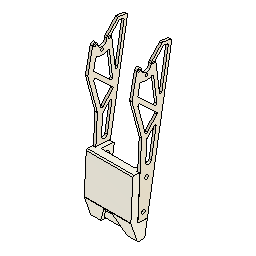
RightArm_7 (Autodesk Fusion 360 archive; units mm, degrees)
design "前腕_16"
Autodesk Fusion 360 part; units mm, degrees
sketch "スケッチ1" plane through (0, 0, 0) normal (1, 0, 0) x (0, 1, 0)
  circle A0 centre (0, 0) radius 4.025
  circle A1 centre (0, 0) radius 6 construction
  circle A2 centre (-6, 0) radius 1.025
  circle A3 centre (0, -6) radius 1.025
  circle A4 centre (6, 0) radius 1.025
  circle A5 centre (-6, 0) radius 1.975
  circle A6 centre (6, 0) radius 1.975
  arc A7 (-7.975, 0) -> (7.975, 0.000024) centre (0, 0) ccw
  line L0 (-7.040069, -110) -> (0.959931, -110)
  line L1 (0.959931, -110) -> (12.959931, -40)
  line L2 (12.959931, -40) -> (7.959931, 0.243509) construction
  circle A8 centre (0, 0) radius 10 construction
  line L3 (-7.936647, 0.387329) -> (-11.936647, -19.612671)
  line L4 (-11.936647, -19.612671) -> (-3.936647, -49.612671)
  line L5 (-3.936647, -49.612671) -> (-7.040069, -110)
  line L6 (9.714999, -38.214272) -> (4.330327, -69.624859)
  line L7 (0.409792, -52.716267) -> (-7.806231, -21.906181)
  line L8 (-7.806231, -21.906181) -> (-5.140514, -8.577594)
  line L9 (9.714999, -38.214272) -> (5.964373, -8.026597)
  arc A9 (-5.140514, -8.577594) -> (5.964373, -8.026597) centre (0, 0) ccw
  line L10 (-0.432003, -69.096168) -> (0.409792, -52.716267)
  arc A10 (-0.432003, -69.096168) -> (4.330327, -69.624859) centre (1.964834, -69.219346) ccw
  circle A11 centre (0.264062, -80) radius 5.754778 construction
  circle A12 centre (-2.400304, -104) radius 4.325705 construction
  circle A13 centre (0.264062, -80) radius 1.55
  circle A14 centre (-2.400304, -104) radius 1.55
  line L11 (12.959931, -40) -> (21.471066, 9.648289)
  line L12 (21.471066, 9.648289) -> (13.586088, 11)
  line L13 (13.586088, 11) -> (4.557732, 1.349254)
  line L14 (18.584601, 7.606643) -> (11.894088, -31.421349)
  line L15 (7.841144, 1.199587) -> (11.894088, -31.421349)
  line L16 (14.491434, 8.308329) -> (7.841144, 1.199587)
  line L17 (9.714999, -38.214272) -> (-0.505264, -49.284806)
  line L18 (8.783943, -43.645432) -> (0.409792, -52.716267)
  line L19 (9.714999, -38.214272) -> (-7.806231, -21.906181)
  line L20 (-7.115191, -18.450978) -> (9.139215, -33.579957)
  line L21 (18.584601, 7.606643) -> (14.491434, 8.308329)
  dimension "d1" = 8.05
  dimension "d2" = 12
  dimension "d3" = 2.05
  dimension "d5" = 110
  dimension "d14" = 20
  dimension "d15" = 4
  dimension "d16" = 20
  dimension "d17" = 5
  dimension "d18" = 70
  dimension "d19" = 30
  dimension "d20" = 8
  dimension "d21" = 8
  dimension "d22" = 12
  dimension "d26" = 3
  dimension "d27" = 4.5
  dimension "d28" = 3.4
  dimension "d29" = 3.5
  dimension "d30" = 4.5
  dimension "d32" = 6
  dimension "d33" = 24
  dimension "d34" = 3.1
  dimension "d35" = 8
  dimension "d36" = 11
  dimension "d38" = 2.5
  dimension "d46" = 3
  dimension "d47" = 3
  dimension "d70" = 2.5
  dimension "d72" = 2.5
  dimension "d73" = 2.4
  constraint coincident A0.centre A1.centre
  constraint concentric A0 A1
  constraint coincident A1 A2.centre
  constraint coincident A1 A3.centre
  constraint coincident A1 A4.centre
  constraint equal A3 A4
  constraint equal A2 A3
  constraint horizontal A0.centre A4.centre
  constraint horizontal A0.centre A2.centre
  constraint vertical A0.centre A3.centre
  constraint concentric A2 A5
  constraint tangent A0 A5
  constraint concentric A4 A6
  constraint tangent A0 A6
  constraint concentric A0 A7
  constraint tangent A5 A7
  constraint tangent A6 L2
  constraint coincident A5 A7.start
  constraint horizontal L0
  constraint concentric A0 A8
  constraint tangent A5 L3
  constraint parallel L2 L9
  constraint parallel L4 L7
  constraint parallel L3 L8
  constraint parallel L1 L6
  constraint parallel L5 L10
  constraint tangent L6 A10
  constraint tangent L10 A10
  constraint tangent L5 A11
  constraint tangent L1 A11
  constraint tangent L5 A12
  constraint tangent L1 A12
  constraint concentric A11 A13
  constraint concentric A12 A14
  constraint equal A13 A14
  constraint collinear L1 L11
  constraint perpendicular L11 L12
  constraint tangent A6 L13
  constraint parallel L11 L14
  constraint parallel L13 L16
  constraint parallel L17 L18
  constraint parallel L19 L20
  constraint parallel L12 L21
  measures "d1" diameter of A0
  measures "d2" diameter of A1
  measures "d3" diameter of A2
  measures "d5" distance of A0.centre L0
  measures "d14" diameter of A8
  measures "d26" distance of L2 L9
  measures "d27" distance of L3 L8
  measures "d28" distance of L4 L7
  measures "d29" distance of L1 L6
  measures "d30" distance of L5 L10
  measures "d34" diameter of A13
  measures "d38" distance of L11 L14
  measures "d46" distance of L17 L18
  measures "d47" distance of L19 L20
  measures "d70" distance of L13 L16
  measures "d72" distance of L12 L21
  measures "d73" radius of A10
extrude "押し出し1" add sketch "スケッチ1" along normal blind 2 contours A0 A5 A6 A7 | A6 | A5 | A5 A6 A7 L0 L1 L3 L4 L5 L11 L12 L13 | L8 L9 L19 L20 | L6 L7 L17 L18 picked at (-4.805093, -3.203034) picked at (7.647164, -0.149042) picked at (-7.65098, -0.098119) picked at (-4.085876, -79.829316) picked at (3.682661, -31.23347) picked at (5.997893, -43.714837) makes body 1
fillet "フィレット1" radius 1 19 edges at (1, 7.841144, 1.199587) (1, 11.894088, -31.421349) (1, 5.964373, -8.026597) (1, -5.140514, -8.577594) (1, -0.505264, -49.284806) (1, 0.409792, -52.716267) (1, 8.783943, -43.645432) (1, -11.936647, -19.612671) (1, -3.936647, -49.612671) (1, 13.586088, 11) (1, 21.471066, 9.648289) (1, 0.959931, -110) (1, -7.040069, -110) (1, 9.139215, -33.579957) (1, -7.115191, -18.450978) (1, -7.806231, -21.906181) (1, 9.714999, -38.214272) (1, 14.491434, 8.308329) (1, 18.584601, 7.606643) on bodies 1
extrude "押し出し2" add 1 faces at (2, -8.409318, -9.624556) along direction (1, 0, 0) blind 2 from surface at 35 on bodies 1 bodies 1 makes body 2
sketch "スケッチ2" plane through (37, 0, 0) normal (-1, 0, 0) x (0, -1, 0)
  arc A0 (5.987358, -110) -> (6.98604, -108.948676) centre (5.987358, -109) ccw
  line L0 (6.98604, -108.948676) -> (3.944718, -49.769715)
  arc A1 (3.977165, -49.460728) -> (3.944718, -49.769715) centre (4.9434, -49.718391) ccw
  line L1 (3.977165, -49.460728) -> (11.876589, -19.837888)
  arc A2 (11.876589, -19.837888) -> (11.890935, -19.384109) centre (10.910354, -19.580225) ccw
  line L2 (11.890935, -19.384109) -> (7.936647, 0.387329)
  arc A3 (7.936647, 0.387329) -> (4.025, 0) centre (6, 0) ccw
  arc A4 (-4.025, 0) -> (4.025, 0) centre (0, 0) ccw
  arc A5 (-4.025, 0) -> (-4.557732, 1.349254) centre (-6, 0) ccw
  line L3 (-4.557732, 1.349254) -> (-13.217964, 10.606498)
  arc A6 (-13.217964, 10.606498) -> (-14.11719, 10.908954) centre (-13.948226, 9.923332) ccw
  line L4 (-14.11719, 10.908954) -> (-20.485444, 9.817253)
  arc A7 (-20.485444, 9.817253) -> (-21.302102, 8.662667) centre (-20.31648, 8.831631) ccw
  line L5 (-21.302102, 8.662667) -> (-1.102394, -109.168964)
  arc A8 (-1.102394, -109.168964) -> (-0.116772, -110) centre (-0.116772, -109) ccw
  line L6 (-0.116772, -110) -> (5.987358, -110)
  line L7 (-14.12331, 7.914828) -> (-8.160973, 1.541465)
  arc A9 (-7.898866, 0.735002) -> (-8.160973, 1.541465) centre (-8.891236, 0.858298) ccw
  line L8 (-7.898866, 0.735002) -> (-11.059631, -24.705056)
  arc A10 (-13.037624, -24.750725) -> (-11.059631, -24.705056) centre (-12.052001, -24.581761) ccw
  line L9 (-13.037624, -24.750725) -> (-18.415637, 6.621021)
  arc A11 (-4.330327, -69.624859) -> (0.432003, -69.096168) centre (-1.964834, -69.219346) ccw
  line L10 (-4.330327, -69.624859) -> (-8.213265, -46.974387)
  arc A12 (-6.492883, -46.127097) -> (-8.213265, -46.974387) centre (-7.227643, -46.805424) ccw
  line L11 (-6.492883, -46.127097) -> (-0.655149, -52.450498)
  arc A13 (-0.391227, -53.0775) -> (-0.655149, -52.450498) centre (-1.389909, -53.128825) ccw
  line L12 (-0.391227, -53.0775) -> (0.432003, -69.096168)
  circle A14 centre (0, -6) radius 1.025
  line L13 (5.400373, -9.876889) -> (7.005667, -17.903357)
  arc A15 (6.706397, -18.831467) -> (7.005667, -17.903357) centre (6.025086, -18.099473) ccw
  line L14 (6.706397, -18.831467) -> (-7.126519, -31.706616)
  arc A16 (-8.8002, -30.851327) -> (-7.126519, -31.706616) centre (-7.80783, -30.974623) ccw
  line L15 (-8.8002, -30.851327) -> (-6.158386, -9.588155)
  arc A17 (-4.696379, -8.828592) -> (-6.158386, -9.588155) centre (-5.166016, -9.711451) ccw
  arc A18 (-4.696379, -8.828592) -> (4.017993, -9.157278) centre (0, 0) ccw
  arc A19 (5.400373, -9.876889) -> (4.017993, -9.157278) centre (4.419792, -10.073005) ccw
  circle A20 centre (6, 0) radius 1.025
  line L16 (-0.727474, -47.94951) -> (-9.039427, -38.946048)
  arc A21 (-8.985979, -37.535728) -> (-9.039427, -38.946048) centre (-8.304667, -38.267721) ccw
  line L17 (-8.985979, -37.535728) -> (5.263716, -24.272656)
  arc A22 (6.911263, -25.262313) -> (5.263716, -24.272656) centre (5.945028, -25.00465) ccw
  line L18 (6.911263, -25.262313) -> (0.973521, -47.528846)
  arc A23 (-0.727474, -47.94951) -> (0.973521, -47.528846) centre (0.007286, -47.271183) ccw
  circle A24 centre (-6, 0) radius 1.025
  circle A25 centre (-0.264062, -80) radius 1.55
  circle A26 centre (2.400304, -104) radius 1.55
  line L19 (-7.302788, -73) -> (5.138567, -73)
  line L20 (5.138567, -73) -> (9.138567, -76)
  line L21 (9.138567, -76) -> (12.825784, -106)
  line L22 (12.825784, -106) -> (8.325784, -141)
  line L23 (8.325784, -141) -> (3.325784, -135)
  line L24 (3.325784, -135) -> (-1.102394, -109.168964)
  circle A27 centre (-0.264062, -80) radius 2.5
  circle A28 centre (2.400304, -104) radius 2.5
  line L25 (-17.598979, 7.775607) -> (-15.022536, 8.217283)
  arc A29 (-14.12331, 7.914828) -> (-15.022536, 8.217283) centre (-14.853572, 7.231661) ccw
  arc A30 (-17.598979, 7.775607) -> (-18.415637, 6.621021) centre (-17.430015, 6.789985) ccw
  dimension "d51" = 25
  dimension "d53" = 3
  dimension "d54" = 4.5
  dimension "d55" = 4
  dimension "d56" = 30
  dimension "d57" = 35
  dimension "d58" = 5
  dimension "d59" = 5
  dimension "d62" = 7
  constraint collinear L5 L24
  constraint horizontal L19
  constraint concentric A25 A27
  constraint concentric A26 A28
  constraint equal A27 A28
  measures "d59" diameter of A27
extrude "押し出し3" add sketch "スケッチ2" along normal up to surface (35 mm away) separate body contours A0 L0 L5 A8 L6 L19 | A0 L0 A8 L6 L20 L21 L22 L23 L24 picked at (-0.871703, -74.50233) picked at (8.159117, -127.333333) makes body 3
sketch "スケッチ3" plane through (2, 0, 0) normal (-1, 0, 0) x (0, -1, 0)
  line L0 (5.138567, -73) -> (-7.302788, -73)
  line L1 (-7.302788, -73) -> (3.325784, -135)
  line L2 (3.325784, -135) -> (8.325784, -141)
  line L3 (8.325784, -141) -> (12.825784, -106)
  line L4 (12.825784, -106) -> (9.138567, -76)
  line L5 (9.138567, -76) -> (5.138567, -73)
  circle A0 centre (-0.264062, -80) radius 2.5
  circle A1 centre (2.400304, -104) radius 2.5
  line L6 (2.724697, -73) -> (6.778563, -105.98314)
  line L7 (6.778563, -105.98314) -> (4.642202, -122.599278)
  line L8 (4.642202, -122.599278) -> (1.298218, -123.172533)
  line L9 (5.138567, -73) -> (-7.302788, -73)
  dimension "d63" = 6
  dimension "d64" = 12
  dimension "d68" = 6
  constraint perpendicular L1 L8
  constraint parallel L3 L7
  constraint parallel L4 L6
  measures "d63" distance of L3 L7
  measures "d68" distance of L4 L6
extrude "押し出し4" cut sketch "スケッチ3" against normal up to surface (25 mm away) from surface at -5 contours L0 L1 L6 L7 L8 L9 picked at (-1.799485, -74.520893) bodies 3
chamfer "面取り1" distance 0.8 angle 45 17 edges at (34.5, 7.302788, -73) (4.5, 7.302788, -73) (19.5, -2.724697, -73) (19.5, -1.298218, -123.172533) (19.5, -8.325784, -141) (2, 1.988502, -104) (2, -5.825784, -138) (2, -10.575784, -123.5) (2, -7.138567, -74.5) (2, 1.08211, -73) (2, -10.982175, -91) (37, 1.08211, -73) (37, 1.988502, -104) (37, -7.138567, -74.5) (37, -10.982175, -91) (37, -10.575784, -123.5) (37, -5.825784, -138) on bodies 3
copy_body "ボディ -> コンポーネント1" bodies 1 removing the originals makes body 4 in component "Component'"
sketch "スケッチ4" plane through (37, 0, 0) normal (-1, 0, 0) x (0, -1, 0)
  arc A0 (5.987358, -110) -> (6.98604, -108.948676) centre (5.987358, -109) ccw
  line L0 (6.98604, -108.948676) -> (3.944718, -49.769715)
  arc A1 (3.977165, -49.460728) -> (3.944718, -49.769715) centre (4.9434, -49.718391) ccw
  line L1 (3.977165, -49.460728) -> (11.876589, -19.837888)
  arc A2 (11.876589, -19.837888) -> (11.890935, -19.384109) centre (10.910354, -19.580225) ccw
  line L2 (11.890935, -19.384109) -> (7.936647, 0.387329)
  arc A3 (7.936647, 0.387329) -> (4.025, 0) centre (6, 0) ccw
  arc A4 (-4.025, 0) -> (4.025, 0) centre (0, 0) ccw
  arc A5 (-4.025, 0) -> (-4.557732, 1.349254) centre (-6, 0) ccw
  line L3 (-4.557732, 1.349254) -> (-13.217964, 10.606498)
  arc A6 (-13.217964, 10.606498) -> (-14.11719, 10.908954) centre (-13.948226, 9.923332) ccw
  line L4 (-14.11719, 10.908954) -> (-20.485444, 9.817253)
  arc A7 (-20.485444, 9.817253) -> (-21.302102, 8.662667) centre (-20.31648, 8.831631) ccw
  line L5 (-21.302102, 8.662667) -> (-1.102394, -109.168964)
  arc A8 (-1.102394, -109.168964) -> (-0.116772, -110) centre (-0.116772, -109) ccw
  line L6 (-0.116772, -110) -> (5.987358, -110)
  circle A9 centre (0, -6) radius 1.025
  circle A10 centre (-0.264062, -80) radius 1.55
  arc A11 (-4.330327, -69.624859) -> (0.432003, -69.096168) centre (-1.964834, -69.219346) ccw
  line L7 (-4.330327, -69.624859) -> (-8.213265, -46.974387)
  arc A12 (-6.492883, -46.127097) -> (-8.213265, -46.974387) centre (-7.227643, -46.805424) ccw
  line L8 (-6.492883, -46.127097) -> (-0.655149, -52.450498)
  arc A13 (-0.391227, -53.0775) -> (-0.655149, -52.450498) centre (-1.389909, -53.128825) ccw
  line L9 (-0.391227, -53.0775) -> (0.432003, -69.096168)
  circle A14 centre (6, 0) radius 1.025
  circle A15 centre (2.400304, -104) radius 1.55
  line L10 (-17.598979, 7.775607) -> (-15.022536, 8.217283)
  arc A16 (-14.12331, 7.914828) -> (-15.022536, 8.217283) centre (-14.853572, 7.231661) ccw
  line L11 (-14.12331, 7.914828) -> (-8.160973, 1.541465)
  arc A17 (-7.898866, 0.735002) -> (-8.160973, 1.541465) centre (-8.891236, 0.858298) ccw
  line L12 (-7.898866, 0.735002) -> (-11.059631, -24.705056)
  arc A18 (-13.037624, -24.750725) -> (-11.059631, -24.705056) centre (-12.052001, -24.581761) ccw
  line L13 (-13.037624, -24.750725) -> (-18.415637, 6.621021)
  arc A19 (-17.598979, 7.775607) -> (-18.415637, 6.621021) centre (-17.430015, 6.789985) ccw
  line L14 (-0.727474, -47.94951) -> (-9.039427, -38.946048)
  arc A20 (-8.985979, -37.535728) -> (-9.039427, -38.946048) centre (-8.304667, -38.267721) ccw
  line L15 (-8.985979, -37.535728) -> (5.263716, -24.272656)
  arc A21 (6.911263, -25.262313) -> (5.263716, -24.272656) centre (5.945028, -25.00465) ccw
  line L16 (6.911263, -25.262313) -> (0.973521, -47.528846)
  arc A22 (-0.727474, -47.94951) -> (0.973521, -47.528846) centre (0.007286, -47.271183) ccw
  line L17 (5.400373, -9.876889) -> (7.005667, -17.903357)
  arc A23 (6.706397, -18.831467) -> (7.005667, -17.903357) centre (6.025086, -18.099473) ccw
  line L18 (6.706397, -18.831467) -> (-7.126519, -31.706616)
  arc A24 (-8.8002, -30.851327) -> (-7.126519, -31.706616) centre (-7.80783, -30.974623) ccw
  line L19 (-8.8002, -30.851327) -> (-6.158386, -9.588155)
  arc A25 (-4.696379, -8.828592) -> (-6.158386, -9.588155) centre (-5.166016, -9.711451) ccw
  arc A26 (-4.696379, -8.828592) -> (4.017993, -9.157278) centre (0, 0) ccw
  arc A27 (5.400373, -9.876889) -> (4.017993, -9.157278) centre (4.419792, -10.073005) ccw
  circle A28 centre (-6, 0) radius 1.025
  circle A29 centre (-0.264062, -80) radius 5.754778 construction
  line L20 (-7.031006, -74.585394) -> (11.179865, -73.649502)
  line L21 (11.179865, -73.649502) -> (12.909897, -107.313001)
  line L22 (12.909897, -107.313001) -> (7.354355, -123.5)
  line L23 (7.354355, -123.5) -> (1.354355, -123.5)
  line L24 (-7.031006, -74.585394) -> (1.354355, -123.5)
  circle A30 centre (5.987358, -109) radius 6 construction
  circle A31 centre (-0.264062, -80) radius 2.4
  circle A32 centre (2.400304, -104) radius 2.4
  dimension "d78" = 123.5
  dimension "d79" = 6
  dimension "d80" = 6
  dimension "d81" = 5
  dimension "d82" = 4.8
  constraint concentric A10 A29
  constraint tangent L5 A29
  constraint perpendicular L0 L20
  constraint tangent A29 L20
  constraint horizontal L23
  constraint parallel L5 L24
  constraint parallel L0 L21
  constraint concentric A0 A30
  constraint tangent L22 A30
  constraint concentric A29 A31
  constraint concentric A15 A32
  constraint equal A31 A32
  measures "d78" distance of A4.centre L23
  measures "d79" distance of L0 L21
  measures "d81" distance of A0 A30
  measures "d82" diameter of A31
extrude "押し出し5" add sketch "スケッチ4" along normal up to surface (35 mm away) separate body contours A0 L0 L5 A8 L6 L20 L24 | A0 L0 A8 L6 L20 L21 L22 L23 L24 picked at (-0.762216, -75.383184) picked at (8.361236, -96.739708) makes body 5
sketch "スケッチ5" plane through (0, 19.25132, -3.300226) normal (0, 0.985622, -0.168964) x (-1, 0, 0)
  line L0 (-2, -121.953185) -> (-2, -72.325038)
  line L1 (-2, -72.325038) -> (-37, -72.325038)
  line L2 (-37, -72.325038) -> (-37, -121.953185)
  line L3 (-37, -121.953185) -> (-2, -121.953185)
  line L4 (-37, -122.966968) -> (-2, -122.966968)
  line L5 (-31, -122.966968) -> (-23.494447, -109.966968)
  line L6 (-23.494447, -109.966968) -> (-15.505553, -109.966968)
  line L7 (-15.505553, -109.966968) -> (-8, -122.966968)
  dimension "d85" = 60
  dimension "d86" = 60
  dimension "d87" = 6
  dimension "d88" = 6
  dimension "d89" = 13
  constraint parallel L3 L6
  measures "d85" angle of L4 L7
  measures "d86" angle of L4 L5
  measures "d89" distance of L4 L6
extrude "押し出し6" cut sketch "スケッチ5" along normal up to surface contours L3 L4 L5 L7 | L3 L5 L6 L7 picked at (-23.138231, -122.629041) picked at (-20.831482, -117.95778) end surface through (37, -12.909897, -107.313001) normal (0, -0.94584347, -0.32462307) offset 0 bodies 5
ref_plane "作業平面1" through (19.5, -0.118541, -98.535805) normal (0, 0.985622, -0.168964) x (0, -0.168964, -0.985622)
sketch "スケッチ6" plane through (0, 16.294454, -2.793335) normal (0, 0.985622, -0.168964) x (0, -0.168964, -0.985622)
  line L0 (122.467471, -8.288385) -> (122.467471, -2)
  line L1 (109.966968, -15.505553) -> (122.467471, -8.288385)
  line L2 (109.966968, -23.494447) -> (109.966968, -15.505553)
  line L3 (122.467471, -30.711615) -> (109.966968, -23.494447)
  line L4 (122.467471, -37) -> (122.467471, -30.711615)
  line L5 (119.467471, -10.020436) -> (119.467471, -28.979564)
  dimension "d94" = 3
  constraint parallel L0 L5
  measures "d94" distance of L0 L5
ref_plane "作業平面2" through (19.5, -8.240439, -114.757254) normal (0, -0.945843, -0.324623) x (0, -0.324623, 0.945843)
sketch "スケッチ7" plane through (0, -42.607427, -14.623301) normal (0, -0.945843, -0.324623) x (0, -0.324623, 0.945843)
  line L0 (-115.110695, -2) -> (-115.110695, -8.206274)
  line L1 (-115.110695, -8.206274) -> (-100.701306, -15.505553)
  line L2 (-100.701306, -15.505553) -> (-100.701306, -23.494447)
  line L3 (-100.701306, -23.494447) -> (-115.110695, -30.793726)
  line L4 (-112.110695, -9.725966) -> (-112.110695, -29.274034)
  dimension "d96" = 3
  constraint vertical L4
loft "ロフト1" add profiles "スケッチ7", "スケッチ6" section 1 contours L1 L2 L3 L4 picked at (-108.307565, -20.831482) section 2 contours L1 L2 L3 L5 picked at (116.300637, -20.831482) bodies 5
sketch "スケッチ8" plane through (0, 19.25132, -3.300226) normal (0, 0.985622, -0.168964) x (-1, 0, 0)
  line L0 (-30.414692, -121.953185) -> (-23.494447, -109.966968)
  line L1 (-23.494447, -109.966968) -> (-15.505553, -109.966968)
  line L2 (-15.505553, -109.966968) -> (-8.585308, -121.953185)
  line L3 (-8.585308, -121.953185) -> (-2, -121.953185)
  line L4 (-2, -121.953185) -> (-2, -72.325038)
  line L5 (-2, -72.325038) -> (-37, -72.325038)
  line L6 (-37, -72.325038) -> (-37, -121.953185)
  line L7 (-37, -121.953185) -> (-30.414692, -121.953185)
  line L8 (-2, -80.355163) -> (-2, -77.255163)
  line L9 (-2, -104.460279) -> (-2, -101.360279)
  line L10 (-37, -80.355163) -> (-37, -77.255163)
  line L11 (-37, -104.460279) -> (-37, -101.360279)
  line L12 (-37, -76.405163) -> (-37, -81.205163)
  line L13 (-37, -100.510279) -> (-37, -105.310279)
  line L14 (-2, -72.325038) -> (-2, -74.47958)
  line L15 (-2, -74.47958) -> (-37, -74.47958) construction
  line L16 (-37, -74.47958) -> (-37, -72.325038)
  line L17 (-37, -72.325038) -> (-2, -72.325038)
  line L18 (-33.6, -72.325038) -> (-5.4, -72.325038)
  line L19 (-5.4, -72.325038) -> (-5.4, -104.951387)
  line L20 (-5.4, -104.951387) -> (-33.6, -104.951387)
  line L21 (-33.6, -104.951387) -> (-33.6, -72.325038)
  line L22 (-37, -107.951387) -> (-2, -107.951387)
  dimension "d97" = 4.8
  dimension "d98" = 3.4
  dimension "d99" = 3.4
  dimension "d100" = 3
  constraint midpoint L10 L12
  constraint parallel L6 L13
  constraint equal L12 L13
  constraint midpoint L11 L13
  constraint horizontal L18
  constraint vertical L19
  constraint horizontal L20
  constraint vertical L21
  measures "d98" distance of L6 L21
  measures "d99" distance of L4 L19
  measures "d100" distance of L20 L22
extrude "押し出し7" cut sketch "スケッチ8" along normal up to surface contours L5 L17 L18 L19 L20 L21 picked at (-14.8, -83.200488) end surface through (37, -11.179865, -73.649502) normal (0, -0.99868204, 0.05132422) offset -8 bodies 5
sketch "スケッチ9" plane through (33.6, 0, 0) normal (-1, 0, 0) x (0, -1, 0)
  line L0 (3.190408, -74.060095) -> (-7.031006, -74.585394)
  line L1 (-7.031006, -74.585394) -> (-1.518334, -106.742649)
  line L2 (-1.518334, -106.742649) -> (1.50084, -106.225076)
  arc A0 (4.692532, -103.288882) -> (1.50084, -106.225076) centre (2.400304, -104) ccw
  line L3 (4.692532, -103.288882) -> (3.190408, -74.060095)
  circle A1 centre (-0.264062, -80) radius 2.4
  circle A2 centre (2.400304, -104) radius 2.4
  circle A3 centre (2.400304, -104) radius 1.55
  line L4 (4.692532, -103.288882) -> (4.753355, -104.472388)
  line L5 (1.50084, -106.225076) -> (3.989514, -105.798447)
  constraint concentric A0 A2
  constraint parallel L3 L4
  constraint parallel L2 L5
extrude "押し出し8" add sketch "スケッチ9" along normal up to surface (28.2 mm away) contours A2 L4 | A2 L5 picked at (4.741762, -104.025781) picked at (2.435653, -106.117154) bodies 5
fillet "フィレット2" radius 1 14 edges at (35.3, 7.031006, -74.585394) (19.5, 1.518334, -106.742649) (19.5, -3.190408, -74.060095) (19.5, -11.179865, -73.649502) (3.7, 7.031006, -74.585394) (19.5, -12.909897, -107.313001) (33.707346, -1.354355, -123.5) (34, -7.354355, -123.5) (5.292654, -1.354355, -123.5) (5, -7.354355, -123.5) (19.5, 0.670882, -111.686118) (19.5, -2.285985, -111.179226) (19.5, -9.91746, -109.870973) (19.5, -12.164162, -109.485824) on bodies 5
fillet "フィレット2" radius 0.6 2 edges at (19.5, -3.891226, -120.543133) (19.5, -6.213709, -120.66247) on bodies 5
fillet "フィレット2" radius 2 1 edges at (19.5, -4.814238, -105.657065) on bodies 5
sketch "スケッチ10" plane through (2, 0, 0) normal (-1, 0, 0) x (0, -1, 0)
  arc A0 (6.640308, -123.5) -> (7.586151, -122.824623) centre (6.640308, -122.5) ccw
  line L0 (7.586151, -122.824623) -> (12.847136, -107.495866)
  arc A1 (12.847136, -107.495866) -> (12.899974, -107.119919) centre (11.901292, -107.171243) ccw
  line L1 (12.899974, -107.119919) -> (11.231189, -74.648184)
  arc A2 (11.231189, -74.648184) -> (10.181183, -73.700826) centre (10.232507, -74.699508) ccw
  line L2 (10.181183, -73.700826) -> (-5.906448, -74.5276)
  arc A3 (-5.906448, -74.5276) -> (-6.840746, -75.695246) centre (-5.855123, -75.526282) ccw
  line L3 (-6.840746, -75.695246) -> (1.211892, -122.668964)
  arc A4 (1.211892, -122.668964) -> (2.197514, -123.5) centre (2.197514, -122.5) ccw
  line L4 (2.197514, -123.5) -> (6.640308, -123.5)
  circle A5 centre (-0.264062, -80) radius 2.4
  circle A6 centre (2.400304, -104) radius 2.4
  arc A7 (5.987358, -110) -> (6.98604, -108.948676) centre (5.987358, -109) ccw
  line L5 (6.98604, -108.948676) -> (3.944718, -49.769715)
  arc A8 (3.977165, -49.460728) -> (3.944718, -49.769715) centre (4.9434, -49.718391) ccw
  line L6 (3.977165, -49.460728) -> (11.876589, -19.837888)
  arc A9 (11.876589, -19.837888) -> (11.890935, -19.384109) centre (10.910354, -19.580225) ccw
  line L7 (11.890935, -19.384109) -> (7.936647, 0.387329)
  arc A10 (7.936647, 0.387329) -> (4.025, 0) centre (6, 0) ccw
  arc A11 (-4.025, 0) -> (4.025, 0) centre (0, 0) ccw
  arc A12 (-4.025, 0) -> (-4.557732, 1.349254) centre (-6, 0) ccw
  line L8 (-4.557732, 1.349254) -> (-13.217964, 10.606498)
  arc A13 (-13.217964, 10.606498) -> (-14.11719, 10.908954) centre (-13.948226, 9.923332) ccw
  line L9 (-14.11719, 10.908954) -> (-20.485444, 9.817253)
  arc A14 (-20.485444, 9.817253) -> (-21.302102, 8.662667) centre (-20.31648, 8.831631) ccw
  line L10 (-21.302102, 8.662667) -> (-1.102394, -109.168964)
  arc A15 (-1.102394, -109.168964) -> (-0.116772, -110) centre (-0.116772, -109) ccw
  line L11 (-0.116772, -110) -> (5.987358, -110)
  circle A16 centre (-6, 0) radius 1.025
  arc A17 (6.706397, -18.831467) -> (7.005667, -17.903357) centre (6.025086, -18.099473) ccw
  line L12 (6.706397, -18.831467) -> (-7.126519, -31.706616)
  arc A18 (-8.8002, -30.851327) -> (-7.126519, -31.706616) centre (-7.80783, -30.974623) ccw
  line L13 (-8.8002, -30.851327) -> (-6.158386, -9.588155)
  arc A19 (-4.696379, -8.828592) -> (-6.158386, -9.588155) centre (-5.166016, -9.711451) ccw
  arc A20 (-4.696379, -8.828592) -> (4.017993, -9.157278) centre (0, 0) ccw
  arc A21 (5.400373, -9.876889) -> (4.017993, -9.157278) centre (4.419792, -10.073005) ccw
  line L14 (5.400373, -9.876889) -> (7.005667, -17.903357)
  arc A22 (-8.985979, -37.535728) -> (-9.039427, -38.946048) centre (-8.304667, -38.267721) ccw
  line L15 (-8.985979, -37.535728) -> (5.263716, -24.272656)
  arc A23 (6.911263, -25.262313) -> (5.263716, -24.272656) centre (5.945028, -25.00465) ccw
  line L16 (6.911263, -25.262313) -> (0.973521, -47.528846)
  arc A24 (-0.727474, -47.94951) -> (0.973521, -47.528846) centre (0.007286, -47.271183) ccw
  line L17 (-0.727474, -47.94951) -> (-9.039427, -38.946048)
  arc A25 (-14.12331, 7.914828) -> (-15.022536, 8.217283) centre (-14.853572, 7.231661) ccw
  line L18 (-14.12331, 7.914828) -> (-8.160973, 1.541465)
  arc A26 (-7.898866, 0.735002) -> (-8.160973, 1.541465) centre (-8.891236, 0.858298) ccw
  line L19 (-7.898866, 0.735002) -> (-11.059631, -24.705056)
  arc A27 (-13.037624, -24.750725) -> (-11.059631, -24.705056) centre (-12.052001, -24.581761) ccw
  line L20 (-13.037624, -24.750725) -> (-18.415637, 6.621021)
  arc A28 (-17.598979, 7.775607) -> (-18.415637, 6.621021) centre (-17.430015, 6.789985) ccw
  line L21 (-17.598979, 7.775607) -> (-15.022536, 8.217283)
  circle A29 centre (2.400304, -104) radius 1.55
  circle A30 centre (6, 0) radius 1.025
  arc A31 (-4.330327, -69.624859) -> (0.432003, -69.096168) centre (-1.964834, -69.219346) ccw
  line L22 (-4.330327, -69.624859) -> (-8.213265, -46.974387)
  arc A32 (-6.492883, -46.127097) -> (-8.213265, -46.974387) centre (-7.227643, -46.805424) ccw
  line L23 (-6.492883, -46.127097) -> (-0.655149, -52.450498)
  arc A33 (-0.391227, -53.0775) -> (-0.655149, -52.450498) centre (-1.389909, -53.128825) ccw
  line L24 (-0.391227, -53.0775) -> (0.432003, -69.096168)
  circle A34 centre (-0.264062, -80) radius 1.55
  circle A35 centre (0, -6) radius 1.025
  arc A36 (4.073788, -49.486495) -> (4.044586, -49.764583) centre (4.9434, -49.718391) ccw
  line L25 (7.085908, -108.943543) -> (4.044586, -49.764583)
  arc A37 (5.987358, -110.1) -> (7.085908, -108.943543) centre (5.987358, -109) ccw
  line L26 (-0.116772, -110.1) -> (5.987358, -110.1)
  arc A38 (-1.200956, -109.18586) -> (-0.116772, -110.1) centre (-0.116772, -109) ccw
  line L27 (-21.400664, 8.645771) -> (-1.200956, -109.18586)
  arc A39 (-20.50234, 9.915816) -> (-21.400664, 8.645771) centre (-20.31648, 8.831631) ccw
  line L28 (-14.134086, 11.007516) -> (-20.50234, 9.915816)
  arc A40 (-13.144938, 10.674815) -> (-14.134086, 11.007516) centre (-13.948226, 9.923332) ccw
  line L29 (-4.484706, 1.417571) -> (-13.144938, 10.674815)
  arc A41 (-3.925, 0) -> (-4.484706, 1.417571) centre (-6, 0) ccw
  arc A42 (-3.925, 0) -> (3.925, 0) centre (0, 0) ccw
  arc A43 (8.034705, 0.406941) -> (3.925, 0) centre (6, 0) ccw
  line L30 (11.988993, -19.364498) -> (8.034705, 0.406941)
  arc A44 (11.973212, -19.863654) -> (11.988993, -19.364498) centre (10.910354, -19.580225) ccw
  line L31 (4.073788, -49.486495) -> (11.973212, -19.863654)
  line L32 (-0.116772, -110.1) -> (-0.942788, -110.1)
  dimension "d109" = 0.1
  constraint tangent A38 L32
  constraint parallel L26 L32
extrude "押し出し9" add sketch "スケッチ10" along normal up to surface (2 mm away) contours A0 L0 A1 L1 A2 L2 L3 A4 L4 L25 A37 L26 L32 picked at (8.424508, -96.671926) bodies 5
fillet "フィレット3" radius 0.6 2 edges at (1, -5.28764, -73.952314) (1, 0.942788, -110.1) on bodies 5
extrude "押し出し10" add 1 faces at (0, -8.434772, -96.871662) along direction (1, 0, 0) up to surface (2 mm away) from surface at 37 on bodies 5 bodies 5
component "Component'" placed x (1, 0, 0) y (0, 1, 0) z (0, 0, 1) at (0, 0, 0)
hidden bodies 3
equation "d88 = d87"
equation "d99 = d98"

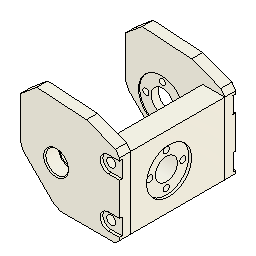
design "肩フレーム_7"
Autodesk Fusion 360 part; units mm, degrees
sketch "スケッチ1" plane through (0, 0, 0) normal (0, 1, 0) x (1, 0, 0)
  line L0 (0, 0) -> (-8, 0)
  line L1 (-8, 0) -> (-8, -26)
  line L2 (-8, -26) -> (0, -26)
  line L3 (0, -26) -> (0, 0)
  line L4 (-4, -22) -> (-4, -4) construction
  line L5 (-4, -13) -> (0, -13) construction
  circle A0 centre (-4, -22) radius 2.325
  circle A1 centre (-4, -4) radius 2.325
  line L6 (-4, -22) -> (-4, -26) construction
  dimension "d1" = 8
  dimension "d2" = 26
  dimension "d4" = 4.65
  dimension "d72" = 4
  constraint horizontal L0
  constraint vertical L1
  constraint horizontal L2
  constraint vertical L3
  constraint coincident L0.start L3.end
  constraint parallel L1 L4
  constraint coincident L4 L5.start
  constraint midpoint L3 L5.end
  constraint horizontal L5
  constraint midpoint L4 L5.start
  constraint coincident L4.start A0.centre
  constraint coincident L4.end A1.centre
  constraint equal A0 A1
  constraint midpoint L2 L6.end
  constraint vertical L6
  measures "d1" distance of L1.end L2.end
  measures "d2" distance of L0.start L2.end
  measures "d4" diameter of A0
  measures "d72" distance of L2 L4.start
extrude "押し出し1" add sketch "スケッチ1" along normal mid plane 34.2 makes body 1
extrude "押し出し2" add sketch "スケッチ1" along normal mid plane 24 contours L0 L1 L2 L3 | A0 | A1 bodies 1
sketch "スケッチ2" plane through (0, 0, 0) normal (1, 0, 0) x (0, 1, 0)
  line L0 (-17.1, 0) -> (17.1, 0)
  line L1 (17.1, 0) -> (17.1, 26)
  line L2 (17.1, 26) -> (-17.1, 26)
  line L3 (-17.1, 26) -> (-17.1, 0)
  circle A0 centre (-3.1, 13) radius 8.15
  line L4 (-3.1, 13) -> (-17.1, 13) construction
  dimension "d9" = 16.3
  dimension "d10" = 14
  constraint coincident A0.centre L4.start
  constraint midpoint L3 L4.end
  constraint horizontal L4
  measures "d9" diameter of A0
  measures "d10" distance of L3 A0.centre
extrude "押し出し3" cut sketch "スケッチ2" against normal blind 1 contours A0 bodies 1
sketch "スケッチ3" plane through (-1, 0, 0) normal (1, 0, 0) x (0, 1, 0)
  circle A0 centre (-3.1, 13) radius 8.15
  circle A1 centre (-3.1, 13) radius 6 construction
  circle A2 centre (-3.1, 19) radius 1.1
  circle A3 centre (-9.1, 13) radius 1.1
  circle A4 centre (-3.1, 7) radius 1.1
  circle A5 centre (2.9, 13) radius 1.1
  circle A6 centre (-3.1, 13) radius 4
  dimension "d14" = 12
  dimension "d15" = 2.2
  dimension "d17" = 360
  dimension "d18" = 8
  constraint concentric A0 A1
  constraint coincident A1 A2.centre
  constraint vertical A0.centre A2.centre
  constraint concentric A1 A6
  measures "d14" diameter of A1
  measures "d15" diameter of A2
  measures "d18" diameter of A6
extrude "押し出し4" cut sketch "スケッチ3" against normal up to surface (7 mm away) contours A2 | A3 | A4 | A5 | A6 bodies 1
sketch "スケッチ4" plane through (-8, 0, 0) normal (-1, 0, 0) x (0, -1, 0)
  circle A0 centre (3.1, 13) radius 4
  circle A1 centre (3.1, 19) radius 1.1
  circle A2 centre (-2.9, 13) radius 1.1
  circle A3 centre (9.1, 13) radius 1.1
  circle A4 centre (3.1, 7) radius 1.1
  line L0 (17.1, 26) -> (-17.1, 26)
  line L1 (-17.1, 26) -> (-17.1, 0)
  line L2 (-17.1, 0) -> (17.1, 0)
  line L3 (17.1, 0) -> (17.1, 26)
  circle A5 centre (3.1, 19) radius 2
  circle A6 centre (-2.9, 13) radius 2
  circle A7 centre (3.1, 7) radius 2
  circle A8 centre (9.1, 13) radius 2
  line L4 (-4.3142, 14.4142) -> (1.6858, 20.4142)
  line L5 (4.5142, 20.4142) -> (10.5142, 14.4142)
  line L6 (10.5142, 11.5858) -> (4.5142, 5.5858)
  line L7 (-4.3142, 11.5858) -> (1.6858, 5.5858)
  dimension "d21" = 4
  dimension "d23" = 360
  constraint concentric A1 A5
  constraint coincident A6 L4.start
  constraint coincident A5 L4.end
  constraint tangent A5 L4
  constraint coincident A5 L5.start
  constraint coincident A8 L5.end
  constraint tangent A8 L5
  constraint coincident A8 L6.start
  constraint coincident A7 L6.end
  constraint tangent A7 L6
  constraint coincident A6 L7.start
  constraint coincident A7 L7.end
  constraint tangent A7 L7
  constraint tangent A6 L7
  constraint tangent A6 L4
  constraint tangent A5 L5
  constraint tangent A8 L6
  measures "d21" diameter of A5
extrude "押し出し5" cut sketch "スケッチ4" against normal blind 1 contours A0 A7 A8 L6 | A0 A5 A8 L5 | A8 | A0 A5 A6 L4 | A5 | A0 A6 A7 L7 | A7 | A6 bodies 1
sketch "スケッチ5" plane through (0, 17.1, 0) normal (0, -1, 0) x (1, 0, 0)
  circle A0 centre (-4, 22) radius 2.325
  circle A1 centre (-4, 4) radius 2.325
  line L0 (0, 0) -> (0, 26)
  line L1 (0, 26) -> (-8, 26)
  line L2 (-8, 26) -> (-8, 0)
  line L3 (-8, 0) -> (0, 0)
  line L4 (-12, 32) -> (-30, 33.2)
  line L5 (-30, 33.2) -> (-36, 28.1654)
  line L6 (-36, 28.1654) -> (-36, 11.8579)
  line L7 (-36, 11.8579) -> (-22.6421, -1.5)
  circle A2 centre (-23, 13) radius 6 construction
  circle A3 centre (-23, 13) radius 4.1
  circle A4 centre (-23, 19) radius 1.1
  circle A5 centre (-29, 13) radius 1.1
  circle A6 centre (-23, 7) radius 1.1
  circle A7 centre (-17, 13) radius 1.1
  line L8 (-33.5, 13) -> (-12.5, 13) construction
  line L9 (-12.5, 13) -> (-12.5, -8) construction
  line L10 (-12.5, -8) -> (-33.5, -8) construction
  line L11 (-33.5, -8) -> (-33.5, 13) construction
  line L12 (-36, -10.5) -> (-10, -10.5) construction
  line L13 (-10, -10.5) -> (-10, 22) construction
  line L14 (-10, 22) -> (-36, 22) construction
  line L15 (-36, 22) -> (-36, -10.5) construction
  line L16 (-8, 0) -> (-8, 26)
  line L17 (0, 0) -> (-8, 0)
  circle A8 centre (-23, 13) radius 8 construction
  circle A9 centre (-4, 22) radius 1.6
  circle A10 centre (-4, 4) radius 1.6
  circle A11 centre (-23, 19) radius 2
  circle A12 centre (-29, 13) radius 2
  line L18 (-30.4142, 14.4142) -> (-24.4142, 20.4142)
  line L19 (-24.4142, 5.5858) -> (-30.4142, 11.5858)
  circle A13 centre (-23, 7) radius 2
  line L20 (-15.5858, 11.5858) -> (-21.5858, 5.5858)
  circle A14 centre (-17, 13) radius 2
  line L21 (-21.5858, 20.4142) -> (-15.5858, 14.4142)
  circle A15 centre (-23, 19) radius 2
  line L22 (0, 0) -> (0, -1.5)
  line L23 (0, -1.5) -> (-22.6421, -1.5)
  line L24 (0, 26) -> (0, 27.5)
  line L25 (0, 27.5) -> (-12, 32)
  circle A16 centre (-4, 4) radius 2.325
  circle A17 centre (-4, 22) radius 2.325
  line L26 (0, 26) -> (0, 0)
  line L27 (0, 0) -> (-8, 0)
  line L28 (-8, 0) -> (-8, 26)
  line L29 (-8, 26) -> (0, 26)
  line L30 (-4, 25) -> (0, 25)
  line L31 (-4, 19) -> (0, 19)
  line L32 (-4, 7) -> (0, 7)
  line L33 (-4, 1) -> (0, 1)
  arc A18 (-4, 25) -> (-4, 19) centre (-4, 22) ccw
  arc A19 (-4, 7) -> (-4, 1) centre (-4, 4) ccw
  dimension "d26" = 12
  dimension "d27" = 8.2
  dimension "d28" = 2.2
  dimension "d30" = 360
  dimension "d31" = 21
  dimension "d32" = 26
  dimension "d33" = 32.5
  dimension "d34" = 2.5
  dimension "d35" = 2.5
  dimension "d37" = 13
  dimension "d38" = 16
  dimension "d40" = 10
  dimension "d42" = 6
  dimension "d43" = 12
  dimension "d44" = 1.2
  dimension "d45" = 18
  dimension "d46" = 3.2
  dimension "d47" = 6
  dimension "d48" = 50
  dimension "d57" = 4
  dimension "d59" = 360
  dimension "d63" = 1.5
  dimension "d102" = 2
  constraint vertical L6
  constraint concentric A2 A3
  constraint coincident A2 A4.centre
  constraint vertical A2.centre A4.centre
  constraint horizontal L8
  constraint vertical L9
  constraint horizontal L10
  constraint vertical L11
  constraint midpoint A2.centre L8
  constraint equal L8 L9
  constraint horizontal L12
  constraint vertical L13
  constraint horizontal L14
  constraint vertical L15
  constraint concentric A2 A8
  constraint coincident L6.end L15
  constraint concentric A0 A9
  constraint concentric A1 A10
  constraint equal A9 A10
  constraint concentric A9 A18
  constraint concentric A10 A19
  constraint equal A18 A19
  constraint concentric A4 A11
  constraint concentric A5 A12
  constraint equal A11 A12
  constraint coincident A12 L18.start
  constraint coincident A11 L18.end
  constraint tangent A11 L18
  constraint tangent A12 L18
  constraint parallel L7 L19
  constraint coincident L0.start L3.end
  constraint perpendicular L17 L22
  constraint perpendicular L9 L23
  constraint coincident L7.end L23.end
  constraint coincident L0.end L1.start
  constraint perpendicular L1 L24
  constraint equal L22 L24
  constraint coincident L0 L30.end
  constraint tangent L30 A18
  constraint perpendicular L0 L30
  constraint coincident L26 L31.end
  constraint tangent L31 A18
  constraint perpendicular L26 L31
  constraint coincident L0 L32.end
  constraint tangent L32 A19
  constraint perpendicular L0 L32
  constraint coincident L26 L33.end
  constraint tangent L33 A19
  constraint perpendicular L26 L33
  measures "d26" diameter of A2
  measures "d27" diameter of A3
  measures "d28" diameter of A4
  measures "d31" distance of L8.start L8.end
  measures "d32" distance of L12.start L12.end
  measures "d33" distance of L12.start L14.end
  measures "d34" distance of L10 L12
  measures "d35" distance of L9 L13
  measures "d37" distance of A2.centre L17
  measures "d38" diameter of A8
  measures "d40" distance of L7 A2.centre
  measures "d42" vertical distance of L0.end L4.start
  measures "d43" horizontal distance of L0.end L4.start
  measures "d44" vertical distance of L4.start L4.end
  measures "d45" horizontal distance of L4.start L4.end
  measures "d46" diameter of A9
  measures "d47" diameter of A18
  measures "d48" angle of L5 L6
  measures "d57" diameter of A11
  measures "d63" distance of L17 L23
  measures "d102" distance of L13 L16
extrude "押し出し6" add sketch "スケッチ5" against normal blind 4 separate body contours A0 A17 | A1 A16 | L0 L1 L2 L3 L16 L17 L26 L27 L28 L29 L30 L31 L32 L33 A18 A19 | L1 L2 L3 L4 L5 L6 L7 L16 L17 L22 L23 L24 L25 L27 L28 L29 | L0 L26 L32 L33 A19 | L0 L26 L30 L31 A18 | A3 A14 | A3 A11 A14 L21 A15 | A3 A13 L20 A14 | A3 A11 A15 | A3 A13 | A3 A11 A12 L18 A15 | A3 A12 L19 A13 | A3 A12 picked at (-18.6059, 13.5457) picked at (-23.0274, 17.3653) picked at (-23.0274, 8.6347) picked at (-27.3709, 13.3372) makes body 2
chamfer "面取り1" distance 1.5 angle 45 4 edges at (-22.6421, 19.1, -1.5) (-36, 19.1, 11.8579) (0, 19.1, 27.5) (0, 19.1, -1.5) on bodies 2
extrude "押し出し10" cut sketch "スケッチ5" along normal blind 1 from surface at -4 contours A0 A17 | A1 A16 | L0 L26 L32 L33 A19 | L0 L26 L30 L31 A18 | A3 A14 | A3 A11 A14 L21 A15 | A3 A13 L20 A14 | A3 A11 A15 | A3 A13 | A3 A11 A12 L18 A15 | A3 A12 L19 A13 | A3 A12 picked at (-18.6059, 13.5457) picked at (-23.0274, 17.3653) picked at (-23.0274, 8.6347) picked at (-27.3709, 13.3372) bodies 2
sketch "スケッチ7" plane through (0, 17.1, 0) normal (0, -1, 0) x (1, 0, 0)
  circle A0 centre (-23, 13) radius 4.1
  circle A1 centre (-23, 19) radius 1.1
  circle A2 centre (-4, 4) radius 1.6
  circle A3 centre (-4, 22) radius 1.6
  circle A4 centre (-17, 13) radius 1.1
  circle A5 centre (-23, 7) radius 1.1
  circle A6 centre (-29, 13) radius 1.1
  line L0 (-1.5, -1.5) -> (0, 0)
  line L1 (0, 0) -> (0, 26)
  line L2 (0, 26) -> (-1.4045, 28.0267)
  line L3 (-1.4045, 28.0267) -> (-12, 32)
  line L4 (-12, 32) -> (-30, 33.2)
  line L5 (-30, 33.2) -> (-36, 28.1654)
  line L6 (-36, 28.1654) -> (-36, 13.3579)
  line L7 (-36, 13.3579) -> (-34.9393, 10.7972)
  line L8 (-34.9393, 10.7972) -> (-23.7028, -0.4393)
  line L9 (-23.7028, -0.4393) -> (-21.1421, -1.5)
  line L10 (-21.1421, -1.5) -> (-1.5, -1.5)
  circle A7 centre (-23, 13) radius 8.25
  dimension "d99" = 16.5
  constraint concentric A0 A7
  measures "d99" diameter of A7
extrude "押し出し15" cut sketch "スケッチ7" against normal blind 0.4 contours A7 bodies 2
sketch "スケッチ6" plane through (0, -17.1, 0) normal (0, -1, 0) x (1, 0, 0)
  circle A0 centre (-4, 4) radius 2.325
  circle A1 centre (-4, 22) radius 2.325
  line L0 (0, 0) -> (0, 26)
  line L1 (0, 26) -> (-8, 26)
  line L2 (-8, 26) -> (-8, 0)
  line L3 (-8, 0) -> (0, 0)
  circle A2 centre (-4, 4) radius 1.6
  circle A3 centre (-4, 22) radius 1.6
  line L4 (-1.5, -1.5) -> (0, 0)
  line L5 (0, 0) -> (0, 26)
  line L6 (0, 26) -> (-1.4045, 28.0267)
  line L7 (-1.4045, 28.0267) -> (-12, 32)
  line L8 (-12, 32) -> (-30, 33.2)
  line L9 (-30, 33.2) -> (-36, 28.1654)
  line L10 (-36, 28.1654) -> (-36, 13.3579)
  line L11 (-36, 13.3579) -> (-34.9393, 10.7972)
  line L12 (-34.9393, 10.7972) -> (-23.7028, -0.4393)
  line L13 (-23.7028, -0.4393) -> (-21.1421, -1.5)
  line L14 (-21.1421, -1.5) -> (-1.5, -1.5)
  circle A4 centre (-23, 13) radius 3.7
  circle A5 centre (-23, 13) radius 6.25
  circle A6 centre (-23, 13) radius 4.1
  circle A7 centre (-23, 13) radius 8.25
  dimension "d77" = 7.4
  dimension "d78" = 8.2
  dimension "d97" = 12.5
  constraint coincident A4.centre A5.centre
  measures "d77" diameter of A4
  measures "d78" diameter of A6
  measures "d97" diameter of A5
extrude "押し出し11" add sketch "スケッチ6" along normal blind 4 separate body contours A0 | A1 | L0 L1 L2 L3 L5 | L1 L2 L3 L4 L6 L7 L8 L9 L10 L11 L12 L13 L14 | A5 | A6 | A7 makes body 3
extrude "押し出し12" add sketch "スケッチ6" against normal blind 3 contours A5 | A6 bodies 3
extrude "押し出し13" cut sketch "スケッチ6" along normal up to surface (5 mm away) from surface at -1 contours A6 bodies 3
chamfer "面取り2" distance 0.4 angle 45 2 edges at (-26.8225, -21.1, 14.4826) (-26.4496, -14.1, 11.662) on bodies 3
chamfer "面取り2" distance 1.4 angle 45 1 edges at (-28.827, -17.1, 10.7399) on bodies 3
extrude "押し出し14" cut 2 faces at (-0.8, 20.1, 22) (-0.8, 20.1, 4) along direction (0, 1, 0) blind 1 start surface through (0, -21.1, 0) normal (0, -1, 0) on bodies 2 bodies 3
